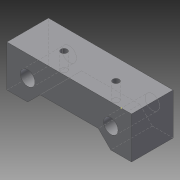
# Autodesk Inventor part: Moving block
Saved by Autodesk Inventor 2015 (Build 190159000, 159)
## iProperties
Created: 2019-01-17
Part Number: Moving block
Material: Generic
Document SubType Name: Modeling
Designer: Toby
Density: 1 g/cm^3
Appearance: Default
Author: Toby
Autodesk Inventor part; units mm, degrees
ref_plane "YZ Plane" through (0, 0, 0) normal (1, 0, 0) x (0, 1, 0)
ref_plane "XZ Plane" through (0, 0, 0) normal (0, 1, 0) x (-1, 0, 0)
ref_plane "XY Plane" through (0, 0, 0) normal (0, 0, 1) x (1, 0, 0)
sketch "Sketch1" plane through (0, 0, 0) normal (0, 0, 1) x (1, 0, 0)
  line L0 (-35.1442, 12.6555) -> (24.8558, 12.6555)
  line L1 (24.8558, 12.6555) -> (24.8558, -7.3445)
  line L2 (24.8558, -7.3445) -> (-35.1442, -7.3445)
  line L3 (-35.1442, -7.3445) -> (-35.1442, 12.6555)
  point P0 (0, 0)
  dimension "d0" = 60
  dimension "d1" = 20
  constraints: 8 end point, 2 parallel, 1 horizontal, 1 perpendicular
  measures "d0" distance of L0.start L0.end
  measures "d1" distance of L2.end L0.start
extrude "Extrusion1" add sketch "Sketch1" along normal blind 20
sketch "Sketch2" plane through (-35.1442, 12.6555, 0) normal (0, 1, 0) x (1, 0, 0)
  line L0 (0, 0) -> (0, -20) projected
  line L1 (60, 0) -> (60, -20) projected
  line L2 (0, 0) -> (60, 0) projected
  circle A0 centre (10, -10) radius 3.5
  circle A1 centre (50, -10) radius 3.5
  point P0 (35.1442, 0)
  dimension "d4" = 40
  dimension "d5" = 10
  dimension "d6" = 10
  dimension "d7" = 10
  dimension "d8" = 7
  dimension "d9" = 7
  constraints: 2 centre point, 2 coincident
  measures "d4" distance of point (50, -10) point (10, -10)
  measures "d5" distance from line of L0 point (10, -10)
  measures "d6" distance from line of L1 point (50, -10)
  measures "d7" distance from line of L2 point (50, -10)
  measures "d8" diameter of A0
  measures "d9" diameter of A1
extrude "Extrusion2" cut sketch "Sketch2" against normal blind 20
sketch "Sketch3" plane through (0, 0, 20) normal (0, 0, 1) x (1, 0, 0)
  line L0 (-35.1442, 12.6555) -> (24.8558, 12.6555) projected
  line L1 (-35.1442, 12.6555) -> (-35.1442, -7.3445) projected
  line L2 (24.8558, -7.3445) -> (24.8558, 12.6555) projected
  point P0 (0, 0)
  point P1 (-17.6442, 2.6555)
  point P2 (7.3558, 2.6555)
  dimension "d12" = 10
  dimension "d13" = 10
  dimension "d14" = 25
  dimension "d15" = 17.5
  dimension "d16" = 17.5
  measures "d12" distance from line of L0 point (-17.644, 2.656)
  measures "d13" distance from line of L0 point (7.356, 2.656)
  measures "d14" distance of point (7.356, 2.656) point (-17.644, 2.656)
  measures "d15" distance from line of L1 point (-17.644, 2.656)
  measures "d16" distance from line of L2 point (7.356, 2.656)
hole "Hole1" at (-17.6442, 2.6555, 20) at (7.3558, 2.6555, 20) direction (0, 0, -1) diameter 3 depth 8 tip angle 118
sketch "Sketch4" plane through (-35.1442, 12.6555, 0) normal (0, 1, 0) x (1, 0, 0)
  line L0 (60, 0) -> (0, 0) projected
  line L1 (16, 0) -> (44, 0)
  line L2 (44, 0) -> (44, -6)
  line L3 (44, -6) -> (16, -6)
  line L4 (16, -6) -> (16, 0)
  line L5 (0, 0) -> (0, -20) projected
  line L6 (60, 0) -> (60, -20) projected
  point P0 (35.1442, 0)
  dimension "d24" = 16
  dimension "d25" = 16
  dimension "d26" = 6
  constraints: 8 end point, 2 parallel, 1 horizontal, 1 perpendicular, 1 point on line
  measures "d24" distance between parallel lines of L5 L4
  measures "d25" distance between parallel lines of L6 L2
  measures "d26" distance between parallel lines of L0 L3
extrude "Extrusion3" cut sketch "Sketch4" against normal blind 20
chamfer "Chamfer1" distance 6 angle 45 2 edges at (8.8558, 2.6555, 0) (-19.1442, 2.6555, 0)
sketch "Sketch5" plane through (-35.1442, 12.6555, 20) normal (0, 1, 0) x (1, 0, 0)
  point P0 (35.1442, 20)
body "Solid1"
